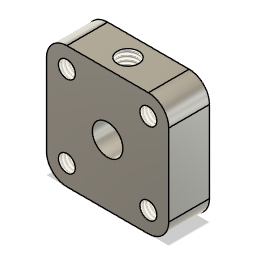
wheel_motor_adapter (Autodesk Fusion 360 design; units mm, degrees)
Autodesk Fusion 360 part; units mm, degrees
sketch "Sketch1" plane through (0, 0, 0) normal (0, 0, 1) x (1, 0, 0)
  circle A0 centre (0, 0) radius 3 construction
  line L0 (12, 12) -> (-12, 12)
  line L1 (-12, 12) -> (-12, -12)
  line L2 (-12, -12) -> (12, -12)
  line L3 (12, -12) -> (12, 12)
  line L4 (12, 12) -> (-12, -12) construction
  line L5 (-12, 12) -> (12, -12) construction
  circle A1 centre (8, 8) radius 1.5 construction
  arc A2 (12, 8) -> (8, 12) centre (8, 8) ccw construction
  circle A3 centre (0, 0) radius 16 construction
  dimension "d1" = 6
  dimension "d2" = 24
  dimension "d3" = 3
  dimension "d4" = 8
  dimension "d23" = 32
  constraint coincident A0.centre A3.centre
  constraint horizontal L0
  constraint perpendicular L0 L1
  constraint parallel L0 L2
  constraint parallel L1 L3
  constraint coincident L4 A0.centre
  constraint coincident L5 A0.centre
  constraint equal L1 L2
  constraint coincident L4 A1.centre
  constraint coincident L3 A2.start
  constraint coincident L0 A2.end
  constraint concentric A1 A2
  constraint tangent L3 A2
  measures "d1" diameter of A0
  measures "d2" distance of L1 L3
  measures "d3" diameter of A1
  measures "d4" horizontal distance of A0.centre A1.centre
  measures "d23" diameter of A3
extrude "Extrude1" add sketch "Sketch1" along normal blind 8
hole "Hole1" at (0, 0, 8) direction (0, 0, -1) diameter 6 end through all
sketch "Sketch2" plane through (0, 0, 8) normal (0, 0, 1) x (1, 0, 0)
  circle A0 centre (0, 0) radius 3
  line L0 (12, -12) -> (12, 12)
  line L1 (12, 12) -> (-12, 12)
  line L2 (-12, 12) -> (-12, -12)
  line L3 (-12, -12) -> (12, -12)
  line L4 (8, 8) -> (-8, 8)
  line L5 (-8, 8) -> (-8, -8)
  line L6 (-8, -8) -> (8, -8)
  line L7 (8, -8) -> (8, 8)
  line L8 (8, 8) -> (-8, -8) construction
  line L9 (-8, 8) -> (8, -8) construction
  dimension "d10" = 16
  constraint horizontal L4
  constraint perpendicular L4 L5
  constraint parallel L4 L6
  constraint parallel L5 L7
  constraint coincident L8 A0.centre
  constraint coincident L9 A0.centre
  constraint coincident A0.centre origin
  constraint equal L5 L6
  measures "d10" distance of L5 L7
hole "Hole2" at (8, 8, 8) at (-8, 8, 8) at (-8, -8, 8) at (8, -8, 8) direction (0, 0, -1) diameter 3.332 end through all
thread "Thread1" "ISO Metric profile 4.0 M4x0.7 M4x0.7 6H" thread offset 0 thread depth 7.4
sketch "Sketch3" plane through (0, 12, 0) normal (0, 1, 0) x (-1, 0, 0)
  line L0 (-12, 0) -> (12, 0)
  line L1 (12, 0) -> (12, 8)
  line L2 (12, 8) -> (-12, 8)
  line L3 (-12, 8) -> (-12, 0)
  line L4 (0, 0) -> (0, 8)
  line L5 (0, 4) -> (-12, 4)
  constraint coincident L4.start origin
  constraint midpoint L2 L4.end
  constraint midpoint L4 L5.start
  constraint midpoint L3 L5.end
hole "Hole3" at (0, 12, 4) direction (0, -1, 0) diameter 4.234 depth 10 tip angle 180
thread "Thread2" "ISO Metric profile 5.0 M5x0.8 M5x0.8 6H" thread offset 0 thread depth 7.4
fillet "Fillet1" radius 4 4 edges at (12, 12, 4) (-12, 12, 4) (12, -12, 4) (-12, -12, 4)
